Autodesk Fusion 360 part; units mm, degrees
(part 2 of 7)
  spline S21 degree 5 poles (-29.1022, 12.0545) (-29.1083, 12.0397) (-29.1203, 12.01) (-29.1375, 11.9653) (-29.159, 11.9055) (-29.1833, 11.8303) (-29.2052, 11.7547) (-29.2246, 11.6787) (-29.2416, 11.6024) (-29.256, 11.5259) (-29.268, 11.4493) (-29.2775, 11.3726) (-29.2844, 11.2962) (-29.2889, 11.22) (-29.2909, 11.1444) (-29.2905, 11.0694) (-29.2877, 10.9953) (-29.2826, 10.9223) (-29.2753, 10.8505) (-29.2659, 10.7801) (-29.2545, 10.7112) (-29.2411, 10.6438) (-29.2258, 10.5781) (-29.2087, 10.5142) (-29.1899, 10.452) (-29.1695, 10.3917) (-29.1478, 10.3334) (-29.125, 10.2775) (-29.1013, 10.2243) (-29.0773, 10.1741) (-29.0531, 10.127) (-29.0289, 10.0831) (-29.005, 10.042) (-28.9815, 10.0035) (-28.9585, 9.967) (-28.9365, 9.9326) (-28.9164, 9.9006) (-28.8995, 9.8722) (-28.8873, 9.8487) (-28.8804, 9.8308) (-28.8783, 9.8185) (-28.8793, 9.8102) (-28.8813, 9.8039) (-28.8835, 9.7977) (-28.8879, 9.7905) (-28.897, 9.7819) (-28.9133, 9.772) (-28.9374, 9.7607) (-28.968, 9.7485) (-29.0034, 9.7354) (-29.0418, 9.7214) (-29.0823, 9.7065) (-29.1244, 9.6903) (-29.1684, 9.6723) (-29.2143, 9.6521) (-29.2622, 9.6295) (-29.3118, 9.6043) (-29.363, 9.5764) (-29.4151, 9.546) (-29.4678, 9.513) (-29.5206, 9.4776) (-29.5734, 9.4397) (-29.6259, 9.3993) (-29.678, 9.3565) (-29.7297, 9.3112) (-29.7807, 9.2635) (-29.8311, 9.2134) (-29.8806, 9.1609) (-29.9291, 9.1061) (-29.9764, 9.049) (-30.0223, 8.9898) (-30.0668, 8.9285) (-30.1096, 8.8654) (-30.1506, 8.8005) (-30.1898, 8.7339) (-30.2269, 8.6658) (-30.262, 8.5963) (-30.295, 8.5255) (-30.3258, 8.4534) (-30.3545, 8.3801) (-30.3809, 8.3056) (-30.4003, 8.2451) (-30.4139, 8.1991) (-30.4225, 8.1683) (-30.4267, 8.1528) knots 0 0 0 0 0 0 0.0125 0.025 0.0375 0.05 0.0625 0.075 0.0875 0.1 0.1125 0.125 0.1375 0.15 0.1625 0.175 0.1875 0.2 0.2125 0.225 0.2375 0.25 0.2625 0.275 0.2875 0.3 0.3125 0.325 0.3375 0.35 0.3625 0.375 0.3875 0.4 0.4125 0.425 0.4375 0.45 0.4625 0.475 0.4875 0.5 0.5125 0.525 0.5375 0.55 0.5625 0.575 0.5875 0.6 0.6125 0.625 0.6375 0.65 0.6625 0.675 0.6875 0.7 0.7125 0.725 0.7375 0.75 0.7625 0.775 0.7875 0.8 0.8125 0.825 0.8375 0.85 0.8625 0.875 0.8875 0.9 0.9125 0.925 0.9375 0.95 0.9625 0.975 0.9875 1 1 1 1 1 1
  spline S22 degree 5 poles (-30.4267, 8.1528) (-30.4308, 8.1373) (-30.4388, 8.1063) (-30.45, 8.0597) (-30.4635, 7.9976) (-30.4778, 7.9199) (-30.4897, 7.8421) (-30.499, 7.7642) (-30.5058, 7.6864) (-30.5102, 7.6086) (-30.512, 7.5311) (-30.5114, 7.4539) (-30.5083, 7.3771) (-30.5028, 7.301) (-30.495, 7.2258) (-30.4848, 7.1515) (-30.4723, 7.0785) (-30.4578, 7.0067) (-30.4412, 6.9365) (-30.4226, 6.8679) (-30.4023, 6.8011) (-30.3802, 6.736) (-30.3565, 6.6729) (-30.3312, 6.6117) (-30.3044, 6.5525) (-30.2764, 6.4954) (-30.2472, 6.4405) (-30.2173, 6.388) (-30.1869, 6.3384) (-30.1565, 6.2917) (-30.1263, 6.2482) (-30.0967, 6.2078) (-30.0676, 6.1702) (-30.0393, 6.135) (-30.0117, 6.1019) (-29.9854, 6.0706) (-29.9613, 6.0416) (-29.9409, 6.0156) (-29.9256, 5.9939) (-29.9165, 5.9771) (-29.9129, 5.9651) (-29.9127, 5.9568) (-29.9139, 5.9502) (-29.9153, 5.9438) (-29.9186, 5.9361) (-29.9265, 5.9264) (-29.9415, 5.9144) (-29.9638, 5.9001) (-29.9926, 5.884) (-30.026, 5.8664) (-30.0623, 5.8476) (-30.1004, 5.8275) (-30.1401, 5.8059) (-30.1813, 5.7823) (-30.2242, 5.7563) (-30.2687, 5.7276) (-30.3147, 5.6961) (-30.3617, 5.6619) (-30.4094, 5.6249) (-30.4574, 5.5853) (-30.5052, 5.5433) (-30.5525, 5.4988) (-30.5993, 5.4519) (-30.6454, 5.4027) (-30.6907, 5.3511) (-30.7351, 5.2971) (-30.7785, 5.2408) (-30.8207, 5.1823) (-30.8616, 5.1216) (-30.9011, 5.0589) (-30.9389, 4.9942) (-30.975, 4.9277) (-31.0092, 4.8595) (-31.0414, 4.7897) (-31.0715, 4.7186) (-31.0994, 4.6463) (-31.1252, 4.5728) (-31.1486, 4.4983) (-31.1698, 4.4228) (-31.1886, 4.3463) (-31.2051, 4.269) (-31.2164, 4.2065) (-31.2239, 4.1592) (-31.2284, 4.1275) (-31.2305, 4.1116) knots 0 0 0 0 0 0 0.0125 0.025 0.0375 0.05 0.0625 0.075 0.0875 0.1 0.1125 0.125 0.1375 0.15 0.1625 0.175 0.1875 0.2 0.2125 0.225 0.2375 0.25 0.2625 0.275 0.2875 0.3 0.3125 0.325 0.3375 0.35 0.3625 0.375 0.3875 0.4 0.4125 0.425 0.4375 0.45 0.4625 0.475 0.4875 0.5 0.5125 0.525 0.5375 0.55 0.5625 0.575 0.5875 0.6 0.6125 0.625 0.6375 0.65 0.6625 0.675 0.6875 0.7 0.7125 0.725 0.7375 0.75 0.7625 0.775 0.7875 0.8 0.8125 0.825 0.8375 0.85 0.8625 0.875 0.8875 0.9 0.9125 0.925 0.9375 0.95 0.9625 0.975 0.9875 1 1 1 1 1 1
  spline S23 degree 5 poles (-31.2305, 4.1116) (-31.2326, 4.0957) (-31.2364, 4.0639) (-31.2415, 4.0163) (-31.2467, 3.9529) (-31.2508, 3.874) (-31.2524, 3.7953) (-31.2515, 3.7169) (-31.2481, 3.6388) (-31.2423, 3.5612) (-31.234, 3.484) (-31.2233, 3.4076) (-31.2102, 3.3319) (-31.1949, 3.2572) (-31.1772, 3.1836) (-31.1574, 3.1113) (-31.1356, 3.0405) (-31.1118, 2.9713) (-31.0861, 2.9038) (-31.0588, 2.8382) (-31.0299, 2.7746) (-30.9995, 2.713) (-30.9678, 2.6535) (-30.9347, 2.5961) (-30.9004, 2.5409) (-30.8651, 2.4879) (-30.8291, 2.4373) (-30.7926, 2.3893) (-30.756, 2.344) (-30.7197, 2.3017) (-30.6842, 2.2624) (-30.6495, 2.2262) (-30.6158, 2.1928) (-30.583, 2.1616) (-30.5514, 2.1324) (-30.5212, 2.1048) (-30.4935, 2.0792) (-30.4699, 2.0561) (-30.452, 2.0365) (-30.4407, 2.0211) (-30.4356, 2.0097) (-30.4343, 2.0014) (-30.4346, 1.9948) (-30.4352, 1.9882) (-30.4375, 1.9801) (-30.4441, 1.9695) (-30.4573, 1.9557) (-30.4776, 1.9386) (-30.504, 1.9188) (-30.5348, 1.897) (-30.5683, 1.8736) (-30.6036, 1.8487) (-30.6401, 1.8221) (-30.6779, 1.7934) (-30.717, 1.762) (-30.7574, 1.7278) (-30.7988, 1.6905) (-30.841, 1.6504) (-30.8835, 1.6075) (-30.9258, 1.5621) (-30.9677, 1.5141) (-31.0089, 1.4639) (-31.0492, 1.4113) (-31.0884, 1.3565) (-31.1266, 1.2994) (-31.1636, 1.2401) (-31.1992, 1.1786) (-31.2334, 1.1151) (-31.2661, 1.0496) (-31.297, 0.9822) (-31.3261, 0.9131) (-31.3532, 0.8424) (-31.3782, 0.7704) (-31.401, 0.6971) (-31.4216, 0.6226) (-31.4398, 0.5472) (-31.4558, 0.471) (-31.4693, 0.3941) (-31.4804, 0.3164) (-31.4891, 0.2382) (-31.4954, 0.1594) (-31.4984, 0.0959) (-31.4996, 0.0481) (-31.5, 0.016) (-31.5, 0) knots 0 0 0 0 0 0 0.0125 0.025 0.0375 0.05 0.0625 0.075 0.0875 0.1 0.1125 0.125 0.1375 0.15 0.1625 0.175 0.1875 0.2 0.2125 0.225 0.2375 0.25 0.2625 0.275 0.2875 0.3 0.3125 0.325 0.3375 0.35 0.3625 0.375 0.3875 0.4 0.4125 0.425 0.4375 0.45 0.4625 0.475 0.4875 0.5 0.5125 0.525 0.5375 0.55 0.5625 0.575 0.5875 0.6 0.6125 0.625 0.6375 0.65 0.6625 0.675 0.6875 0.7 0.7125 0.725 0.7375 0.75 0.7625 0.775 0.7875 0.8 0.8125 0.825 0.8375 0.85 0.8625 0.875 0.8875 0.9 0.9125 0.925 0.9375 0.95 0.9625 0.975 0.9875 1 1 1 1 1 1
  spline S24 degree 5 poles (-31.5, 0) (-31.5, -0.016) (-31.4996, -0.0481) (-31.4984, -0.0959) (-31.4954, -0.1594) (-31.4891, -0.2382) (-31.4804, -0.3164) (-31.4693, -0.3941) (-31.4558, -0.471) (-31.4398, -0.5472) (-31.4216, -0.6226) (-31.401, -0.697) (-31.3781, -0.7704) (-31.3531, -0.8424) (-31.326, -0.9131) (-31.297, -0.9822) (-31.266, -1.0496) (-31.2334, -1.1151) (-31.1992, -1.1786) (-31.1636, -1.2401) (-31.1266, -1.2994) (-31.0884, -1.3565) (-31.0492, -1.4113) (-31.0089, -1.4639) (-30.9677, -1.5141) (-30.9258, -1.5621) (-30.8835, -1.6075) (-30.841, -1.6504) (-30.7988, -1.6906) (-30.7574, -1.7278) (-30.717, -1.762) (-30.6779, -1.7934) (-30.6401, -1.8221) (-30.6036, -1.8487) (-30.5683, -1.8736) (-30.5348, -1.897) (-30.504, -1.9188) (-30.4776, -1.9386) (-30.4573, -1.9557) (-30.4441, -1.9695) (-30.4375, -1.9801) (-30.4352, -1.9882) (-30.4346, -1.9948) (-30.4343, -2.0014) (-30.4356, -2.0097) (-30.4407, -2.0211) (-30.452, -2.0365) (-30.4699, -2.0561) (-30.4935, -2.0792) (-30.5212, -2.1048) (-30.5514, -2.1324) (-30.583, -2.1616) (-30.6158, -2.1928) (-30.6495, -2.2262) (-30.6842, -2.2624) (-30.7197, -2.3017) (-30.756, -2.344) (-30.7926, -2.3893) (-30.8291, -2.4373) (-30.8652, -2.4879) (-30.9004, -2.5409) (-30.9347, -2.5961) (-30.9677, -2.6535) (-30.9995, -2.713) (-31.0299, -2.7746) (-31.0588, -2.8382) (-31.0862, -2.9038) (-31.1118, -2.9713) (-31.1356, -3.0405) (-31.1575, -3.1113) (-31.1773, -3.1836) (-31.1949, -3.2572) (-31.2103, -3.3319) (-31.2233, -3.4076) (-31.234, -3.484) (-31.2423, -3.5612) (-31.2481, -3.6388) (-31.2515, -3.7169) (-31.2524, -3.7953) (-31.2508, -3.874) (-31.2467, -3.9529) (-31.2415, -4.0163) (-31.2364, -4.0639) (-31.2326, -4.0957) (-31.2305, -4.1116) knots 0 0 0 0 0 0 0.0125 0.025 0.0375 0.05 0.0625 0.075 0.0875 0.1 0.1125 0.125 0.1375 0.15 0.1625 0.175 0.1875 0.2 0.2125 0.225 0.2375 0.25 0.2625 0.275 0.2875 0.3 0.3125 0.325 0.3375 0.35 0.3625 0.375 0.3875 0.4 0.4125 0.425 0.4375 0.45 0.4625 0.475 0.4875 0.5 0.5125 0.525 0.5375 0.55 0.5625 0.575 0.5875 0.6 0.6125 0.625 0.6375 0.65 0.6625 0.675 0.6875 0.7 0.7125 0.725 0.7375 0.75 0.7625 0.775 0.7875 0.8 0.8125 0.825 0.8375 0.85 0.8625 0.875 0.8875 0.9 0.9125 0.925 0.9375 0.95 0.9625 0.975 0.9875 1 1 1 1 1 1
  spline S25 degree 5 poles (-31.2305, -4.1116) (-31.2284, -4.1275) (-31.2239, -4.1592) (-31.2165, -4.2065) (-31.2051, -4.269) (-31.1886, -4.3463) (-31.1698, -4.4228) (-31.1486, -4.4983) (-31.1252, -4.5728) (-31.0994, -4.6463) (-31.0715, -4.7186) (-31.0413, -4.7897) (-31.0091, -4.8595) (-30.9749, -4.9276) (-30.9389, -4.9942) (-30.901, -5.0589) (-30.8616, -5.1216) (-30.8207, -5.1823) (-30.7785, -5.2408) (-30.7351, -5.2971) (-30.6907, -5.3511) (-30.6454, -5.4027) (-30.5993, -5.452) (-30.5525, -5.4988) (-30.5052, -5.5433) (-30.4574, -5.5853) (-30.4094, -5.6249) (-30.3617, -5.6619) (-30.3147, -5.6961) (-30.2687, -5.7276) (-30.2242, -5.7563) (-30.1813, -5.7823) (-30.1401, -5.8059) (-30.1004, -5.8275) (-30.0623, -5.8476) (-30.026, -5.8664) (-29.9926, -5.884) (-29.9638, -5.9001) (-29.9415, -5.9144) (-29.9265, -5.9264) (-29.9186, -5.9361) (-29.9153, -5.9438) (-29.9139, -5.9502) (-29.9127, -5.9568) (-29.9129, -5.9651) (-29.9165, -5.9771) (-29.9257, -5.9939) (-29.9409, -6.0156) (-29.9613, -6.0416) (-29.9854, -6.0706) (-30.0117, -6.1019) (-30.0393, -6.135) (-30.0676, -6.1702) (-30.0967, -6.2078) (-30.1263, -6.2482) (-30.1565, -6.2917) (-30.1869, -6.3384) (-30.2173, -6.3881) (-30.2472, -6.4405) (-30.2764, -6.4954) (-30.3044, -6.5525) (-30.3312, -6.6117) (-30.3565, -6.6729) (-30.3802, -6.736) (-30.4023, -6.8011) (-30.4226, -6.8679) (-30.4412, -6.9365) (-30.4578, -7.0067) (-30.4724, -7.0785) (-30.4848, -7.1515) (-30.495, -7.2258) (-30.5029, -7.3011) (-30.5084, -7.3771) (-30.5115, -7.4539) (-30.5121, -7.5311) (-30.5102, -7.6086) (-30.5058, -7.6864) (-30.499, -7.7642) (-30.4896, -7.8421) (-30.4778, -7.9199) (-30.4634, -7.9976) (-30.45, -8.0597) (-30.4388, -8.1063) (-30.4308, -8.1373) (-30.4267, -8.1528) knots 0 0 0 0 0 0 0.0125 0.025 0.0375 0.05 0.0625 0.075 0.0875 0.1 0.1125 0.125 0.1375 0.15 0.1625 0.175 0.1875 0.2 0.2125 0.225 0.2375 0.25 0.2625 0.275 0.2875 0.3 0.3125 0.325 0.3375 0.35 0.3625 0.375 0.3875 0.4 0.4125 0.425 0.4375 0.45 0.4625 0.475 0.4875 0.5 0.5125 0.525 0.5375 0.55 0.5625 0.575 0.5875 0.6 0.6125 0.625 0.6375 0.65 0.6625 0.675 0.6875 0.7 0.7125 0.725 0.7375 0.75 0.7625 0.775 0.7875 0.8 0.8125 0.825 0.8375 0.85 0.8625 0.875 0.8875 0.9 0.9125 0.925 0.9375 0.95 0.9625 0.975 0.9875 1 1 1 1 1 1
  spline S26 degree 5 poles (-30.4267, -8.1528) (-30.4225, -8.1683) (-30.4139, -8.1991) (-30.4003, -8.2451) (-30.3809, -8.3056) (-30.3545, -8.3801) (-30.3259, -8.4534) (-30.295, -8.5255) (-30.262, -8.5963) (-30.2269, -8.6658) (-30.1897, -8.7339) (-30.1506, -8.8005) (-30.1096, -8.8654) (-30.0668, -8.9285) (-30.0223, -8.9898) (-29.9763, -9.049) (-29.929, -9.106) (-29.8806, -9.1609) (-29.8311, -9.2134) (-29.7807, -9.2635) (-29.7297, -9.3113) (-29.678, -9.3565) (-29.6259, -9.3993) (-29.5734, -9.4397) (-29.5206, -9.4776) (-29.4678, -9.513) (-29.4151, -9.546) (-29.363, -9.5764) (-29.3118, -9.6043) (-29.2621, -9.6295) (-29.2143, -9.6521) (-29.1684, -9.6723) (-29.1244, -9.6903) (-29.0823, -9.7065) (-29.0418, -9.7214) (-29.0034, -9.7354) (-28.968, -9.7485) (-28.9374, -9.7607) (-28.9133, -9.772) (-28.897, -9.7819) (-28.8879, -9.7905) (-28.8835, -9.7977) (-28.8813, -9.8039) (-28.8793, -9.8102) (-28.8783, -9.8185) (-28.8804, -9.8308) (-28.8873, -9.8487) (-28.8995, -9.8722) (-28.9164, -9.9006) (-28.9365, -9.9326) (-28.9585, -9.967) (-28.9815, -10.0035) (-29.005, -10.042) (-29.0289, -10.0831) (-29.0531, -10.127) (-29.0773, -10.1741) (-29.1014, -10.2243) (-29.125, -10.2775) (-29.1478, -10.3334) (-29.1695, -10.3917) (-29.1899, -10.452) (-29.2087, -10.5142) (-29.2258, -10.5781) (-29.2411, -10.6438) (-29.2545, -10.7112) (-29.2659, -10.7801) (-29.2754, -10.8505) (-29.2827, -10.9223) (-29.2878, -10.9954) (-29.2905, -11.0694) (-29.291, -11.1444) (-29.289, -11.22) (-29.2845, -11.2962) (-29.2775, -11.3727) (-29.268, -11.4493) (-29.256, -11.5259) (-29.2416, -11.6024) (-29.2246, -11.6787) (-29.2052, -11.7547) (-29.1833, -11.8303) (-29.1589, -11.9055) (-29.1375, -11.9653) (-29.1203, -12.01) (-29.1083, -12.0397) (-29.1022, -12.0545) knots 0 0 0 0 0 0 0.0125 0.025 0.0375 0.05 0.0625 0.075 0.0875 0.1 0.1125 0.125 0.1375 0.15 0.1625 0.175 0.1875 0.2 0.2125 0.225 0.2375 0.25 0.2625 0.275 0.2875 0.3 0.3125 0.325 0.3375 0.35 0.3625 0.375 0.3875 0.4 0.4125 0.425 0.4375 0.45 0.4625 0.475 0.4875 0.5 0.5125 0.525 0.5375 0.55 0.5625 0.575 0.5875 0.6 0.6125 0.625 0.6375 0.65 0.6625 0.675 0.6875 0.7 0.7125 0.725 0.7375 0.75 0.7625 0.775 0.7875 0.8 0.8125 0.825 0.8375 0.85 0.8625 0.875 0.8875 0.9 0.9125 0.925 0.9375 0.95 0.9625 0.975 0.9875 1 1 1 1 1 1
  spline S27 degree 5 poles (-29.1022, -12.0545) (-29.096, -12.0693) (-29.0835, -12.0988) (-29.0641, -12.1426) (-29.0369, -12.2001) (-29.001, -12.2705) (-28.963, -12.3394) (-28.923, -12.4068) (-28.8811, -12.4728) (-28.8372, -12.5371) (-28.7915, -12.5997) (-28.744, -12.6606) (-28.6948, -12.7196) (-28.6441, -12.7766) (-28.5921, -12.8315) (-28.5388, -12.8842) (-28.4844, -12.9347) (-28.4292, -12.9827) (-28.3733, -13.0283) (-28.3168, -13.0714) (-28.26, -13.1121) (-28.2029, -13.1502) (-28.1456, -13.1859) (-28.0883, -13.219) (-28.031, -13.2497) (-27.974, -13.278) (-27.9174, -13.3038) (-27.8618, -13.3271) (-27.8075, -13.3481) (-27.7549, -13.3666) (-27.7045, -13.3828) (-27.6564, -13.3968) (-27.6104, -13.4089) (-27.5665, -13.4195) (-27.5245, -13.429) (-27.4846, -13.4378) (-27.4477, -13.4462) (-27.4158, -13.4543) (-27.3905, -13.4623) (-27.373, -13.47) (-27.3628, -13.4773) (-27.3576, -13.4839) (-27.3545, -13.4898) (-27.3517, -13.4958) (-27.3497, -13.5039) (-27.3501, -13.5164) (-27.3546, -13.535) (-27.3637, -13.5599) (-27.3767, -13.5903) (-27.3924, -13.6246) (-27.4098, -13.6616) (-27.4278, -13.7007) (-27.4462, -13.742) (-27.4645, -13.7858) (-27.4827, -13.8325) (-27.5005, -13.8824) (-27.5178, -13.9354) (-27.5343, -13.9912) (-27.5496, -14.0496) (-27.5636, -14.1101) (-27.5759, -14.1726) (-27.5864, -14.2367) (-27.595, -14.3024) (-27.6016, -14.3695) (-27.6061, -14.438) (-27.6085, -14.5079) (-27.6086, -14.5789) (-27.6065, -14.651) (-27.602, -14.7241) (-27.5951, -14.7979) (-27.5857, -14.8723) (-27.5739, -14.947) (-27.5595, -15.0219) (-27.5426, -15.0968) (-27.5232, -15.1716) (-27.5013, -15.246) (-27.477, -15.32) (-27.4502, -15.3934) (-27.4211, -15.4662) (-27.3895, -15.5382) (-27.3555, -15.6096) (-27.3264, -15.6661) (-27.3035, -15.7082) (-27.2878, -15.7361) (-27.2798, -15.75) knots 0 0 0 0 0 0 0.0125 0.025 0.0375 0.05 0.0625 0.075 0.0875 0.1 0.1125 0.125 0.1375 0.15 0.1625 0.175 0.1875 0.2 0.2125 0.225 0.2375 0.25 0.2625 0.275 0.2875 0.3 0.3125 0.325 0.3375 0.35 0.3625 0.375 0.3875 0.4 0.4125 0.425 0.4375 0.45 0.4625 0.475 0.4875 0.5 0.5125 0.525 0.5375 0.55 0.5625 0.575 0.5875 0.6 0.6125 0.625 0.6375 0.65 0.6625 0.675 0.6875 0.7 0.7125 0.725 0.7375 0.75 0.7625 0.775 0.7875 0.8 0.8125 0.825 0.8375 0.85 0.8625 0.875 0.8875 0.9 0.9125 0.925 0.9375 0.95 0.9625 0.975 0.9875 1 1 1 1 1 1
  spline S28 degree 5 poles (-27.2798, -15.75) (-27.2717, -15.7639) (-27.2555, -15.7915) (-27.2305, -15.8323) (-27.1961, -15.8858) (-27.1513, -15.9509) (-27.1046, -16.0143) (-27.0562, -16.0759) (-27.006, -16.1358) (-26.9541, -16.1938) (-26.9006, -16.25) (-26.8455, -16.3041) (-26.7891, -16.3562) (-26.7314, -16.4061) (-26.6726, -16.4538) (-26.6129, -16.4991) (-26.5524, -16.542) (-26.4914, -16.5824) (-26.43, -16.6203) (-26.3684, -16.6557) (-26.3067, -16.6886) (-26.2451, -16.7189) (-26.1837, -16.7468) (-26.1226, -16.7722) (-26.0618, -16.7951) (-26.0015, -16.8157) (-25.9421, -16.8339) (-25.8839, -16.8498) (-25.8273, -16.8635) (-25.7728, -16.875) (-25.7207, -16.8844) (-25.6711, -16.892) (-25.624, -16.8981) (-25.5791, -16.9028) (-25.5362, -16.9068) (-25.4954, -16.9103) (-25.4578, -16.9138) (-25.4251, -16.9177) (-25.399, -16.9223) (-25.3806, -16.9277) (-25.3696, -16.9336) (-25.3635, -16.9394) (-25.3597, -16.9448) (-25.3562, -16.9504) (-25.3531, -16.9582) (-25.3519, -16.9707) (-25.3539, -16.9897) (-25.3597, -17.0156) (-25.3686, -17.0474) (-25.3797, -17.0834) (-25.3921, -17.1224) (-25.4049, -17.1636) (-25.4177, -17.2069) (-25.4301, -17.2527) (-25.442, -17.3014) (-25.4532, -17.3532) (-25.4635, -17.4079) (-25.4725, -17.4654) (-25.4801, -17.5253) (-25.486, -17.5872) (-25.4901, -17.6507) (-25.4921, -17.7157) (-25.4921, -17.7819) (-25.4899, -17.8493) (-25.4854, -17.9178) (-25.4786, -17.9874) (-25.4695, -18.0578) (-25.458, -18.1291) (-25.444, -18.2009) (-25.4275, -18.2732) (-25.4085, -18.3457) (-25.387, -18.4182) (-25.363, -18.4906) (-25.3364, -18.5627) (-25.3074, -18.6343) (-25.276, -18.7052) (-25.2423, -18.7754) (-25.2061, -18.8447) (-25.1677, -18.913) (-25.127, -18.9804) (-25.084, -19.0467) (-25.0478, -19.0989) (-25.0196, -19.1376) (-25.0004, -19.1632) (-24.9906, -19.176) knots 0 0 0 0 0 0 0.0125 0.025 0.0375 0.05 0.0625 0.075 0.0875 0.1 0.1125 0.125 0.1375 0.15 0.1625 0.175 0.1875 0.2 0.2125 0.225 0.2375 0.25 0.2625 0.275 0.2875 0.3 0.3125 0.325 0.3375 0.35 0.3625 0.375 0.3875 0.4 0.4125 0.425 0.4375 0.45 0.4625 0.475 0.4875 0.5 0.5125 0.525 0.5375 0.55 0.5625 0.575 0.5875 0.6 0.6125 0.625 0.6375 0.65 0.6625 0.675 0.6875 0.7 0.7125 0.725 0.7375 0.75 0.7625 0.775 0.7875 0.8 0.8125 0.825 0.8375 0.85 0.8625 0.875 0.8875 0.9 0.9125 0.925 0.9375 0.95 0.9625 0.975 0.9875 1 1 1 1 1 1
  spline S29 degree 5 poles (-24.9906, -19.176) (-24.9808, -19.1887) (-24.9611, -19.2139) (-24.931, -19.2512) (-24.8899, -19.2997) (-24.837, -19.3584) (-24.7825, -19.4151) (-24.7264, -19.4699) (-24.6688, -19.5227) (-24.6098, -19.5735) (-24.5494, -19.6222) (-24.4877, -19.6687) (-24.425, -19.713) (-24.3613, -19.7549) (-24.2968, -19.7945) (-24.2316, -19.8316) (-24.1661, -19.8662) (-24.1003, -19.8983) (-24.0345, -19.9279) (-23.9688, -19.955) (-23.9034, -19.9795) (-23.8384, -20.0016) (-23.7738, -20.0212) (-23.7099, -20.0384) (-23.6466, -20.0532) (-23.5842, -20.0657) (-23.5229, -20.076) (-23.4631, -20.0842) (-23.4052, -20.0903) (-23.3497, -20.0946) (-23.2968, -20.0972) (-23.2466, -20.0983) (-23.1992, -20.0981) (-23.154, -20.097) (-23.1109, -20.0953) (-23.0701, -20.0934) (-23.0324, -20.092) (-22.9994, -20.0916) (-22.9729, -20.0928) (-22.9539, -20.0957) (-22.9422, -20.1001) (-22.9355, -20.1051) (-22.931, -20.11) (-22.9268, -20.1151) (-22.9227, -20.1224) (-22.9199, -20.1346) (-22.9194, -20.1537) (-22.9217, -20.1801) (-22.9264, -20.2128) (-22.9328, -20.25) (-22.9399, -20.2902) (-22.9472, -20.3327) (-22.9542, -20.3774) (-22.9606, -20.4244) (-22.9661, -20.4742) (-22.9704, -20.527) (-22.9735, -20.5827) (-22.9749, -20.6409) (-22.9746, -20.7012) (-22.9724, -20.7633) (-22.9681, -20.8268) (-22.9617, -20.8915) (-22.953, -20.9571) (-22.942, -21.0237) (-22.9286, -21.091) (-22.9128, -21.1591) (-22.8946, -21.2278) (-22.8739, -21.2969) (-22.8506, -21.3663) (-22.8248, -21.4358) (-22.7966, -21.5052) (-22.7657, -21.5743) (-22.7325, -21.643) (-22.6968, -21.711) (-22.6587, -21.7782) (-22.6183, -21.8444) (-22.5756, -21.9095) (-22.5308, -21.9735) (-22.4838, -22.0362) (-22.4346, -22.0977) (-22.3833, -22.1579) (-22.3406, -22.2049) (-22.3076, -22.2396) (-22.2852, -22.2625) (-22.2739, -22.2739) knots 0 0 0 0 0 0 0.0125 0.025 0.0375 0.05 0.0625 0.075 0.0875 0.1 0.1125 0.125 0.1375 0.15 0.1625 0.175 0.1875 0.2 0.2125 0.225 0.2375 0.25 0.2625 0.275 0.2875 0.3 0.3125 0.325 0.3375 0.35 0.3625 0.375 0.3875 0.4 0.4125 0.425 0.4375 0.45 0.4625 0.475 0.4875 0.5 0.5125 0.525 0.5375 0.55 0.5625 0.575 0.5875 0.6 0.6125 0.625 0.6375 0.65 0.6625 0.675 0.6875 0.7 0.7125 0.725 0.7375 0.75 0.7625 0.775 0.7875 0.8 0.8125 0.825 0.8375 0.85 0.8625 0.875 0.8875 0.9 0.9125 0.925 0.9375 0.95 0.9625 0.975 0.9875 1 1 1 1 1 1
  spline S30 degree 5 poles (-22.2739, -22.2739) (-22.2625, -22.2852) (-22.2396, -22.3076) (-22.2049, -22.3406) (-22.1579, -22.3833) (-22.0977, -22.4346) (-22.0363, -22.4838) (-21.9735, -22.5308) (-21.9095, -22.5756) (-21.8444, -22.6183) (-21.7781, -22.6587) (-21.7109, -22.6967) (-21.643, -22.7324) (-21.5743, -22.7657) (-21.5052, -22.7965) (-21.4358, -22.8248) (-21.3663, -22.8506) (-21.2969, -22.8738) (-21.2278, -22.8946) (-21.1591, -22.9128) (-21.091, -22.9286) (-21.0237, -22.942) (-20.9571, -22.953) (-20.8915, -22.9617) (-20.8268, -22.9681) (-20.7633, -22.9724) (-20.7012, -22.9746) (-20.6409, -22.9749) (-20.5827, -22.9735) (-20.527, -22.9704) (-20.4742, -22.9661) (-20.4244, -22.9606) (-20.3774, -22.9542) (-20.3327, -22.9472) (-20.2902, -22.9399) (-20.25, -22.9328) (-20.2128, -22.9264) (-20.1801, -22.9217) (-20.1537, -22.9194) (-20.1345, -22.9199) (-20.1224, -22.9227) (-20.1151, -22.9268) (-20.11, -22.931) (-20.1051, -22.9355) (-20.1001, -22.9422) (-20.0957, -22.9539) (-20.0928, -22.9729) (-20.0916, -22.9994) (-20.092, -23.0324) (-20.0934, -23.0701) (-20.0953, -23.1109) (-20.097, -23.154) (-20.0981, -23.1992) (-20.0983, -23.2467) (-20.0972, -23.2968) (-20.0946, -23.3497) (-20.0903, -23.4052) (-20.0842, -23.4631) (-20.076, -23.5229) (-20.0657, -23.5842) (-20.0532, -23.6466) (-20.0384, -23.7099) (-20.0212, -23.7738) (-20.0016, -23.8384) (-19.9795, -23.9034) (-19.955, -23.9688) (-19.9279, -24.0345) (-19.8984, -24.1004) (-19.8663, -24.1661) (-19.8316, -24.2317) (-19.7945, -24.2968) (-19.755, -24.3613) (-19.713, -24.425) (-19.6687, -24.4878) (-19.6222, -24.5494) (-19.5735, -24.6098) (-19.5227, -24.6688) (-19.4699, -24.7264) (-19.4151, -24.7824) (-19.3583, -24.837) (-19.2996, -24.8899) (-19.2511, -24.931) (-19.2139, -24.9611) (-19.1887, -24.9808) (-19.176, -24.9906) knots 0 0 0 0 0 0 0.0125 0.025 0.0375 0.05 0.0625 0.075 0.0875 0.1 0.1125 0.125 0.1375 0.15 0.1625 0.175 0.1875 0.2 0.2125 0.225 0.2375 0.25 0.2625 0.275 0.2875 0.3 0.3125 0.325 0.3375 0.35 0.3625 0.375 0.3875 0.4 0.4125 0.425 0.4375 0.45 0.4625 0.475 0.4875 0.5 0.5125 0.525 0.5375 0.55 0.5625 0.575 0.5875 0.6 0.6125 0.625 0.6375 0.65 0.6625 0.675 0.6875 0.7 0.7125 0.725 0.7375 0.75 0.7625 0.775 0.7875 0.8 0.8125 0.825 0.8375 0.85 0.8625 0.875 0.8875 0.9 0.9125 0.925 0.9375 0.95 0.9625 0.975 0.9875 1 1 1 1 1 1
  spline S31 degree 5 poles (-19.176, -24.9906) (-19.1632, -25.0004) (-19.1376, -25.0196) (-19.0989, -25.0478) (-19.0467, -25.084) (-18.9804, -25.127) (-18.913, -25.1677) (-18.8447, -25.2062) (-18.7754, -25.2423) (-18.7052, -25.276) (-18.6343, -25.3074) (-18.5627, -25.3364) (-18.4906, -25.3629) (-18.4182, -25.387) (-18.3457, -25.4085) (-18.2732, -25.4275) (-18.2009, -25.444) (-18.1291, -25.4579) (-18.0578, -25.4695) (-17.9874, -25.4786) (-17.9178, -25.4854) (-17.8493, -25.4899) (-17.7819, -25.4921) (-17.7157, -25.4922) (-17.6507, -25.4901) (-17.5872, -25.486) (-17.5253, -25.4801) (-17.4654, -25.4725) (-17.4079, -25.4635) (-17.3532, -25.4532) (-17.3014, -25.442) (-17.2527, -25.4301) (-17.2069, -25.4177) (-17.1636, -25.4049) (-17.1224, -25.3921) (-17.0834, -25.3797) (-17.0474, -25.3686) (-17.0156, -25.3597) (-16.9897, -25.3539) (-16.9707, -25.3519) (-16.9582, -25.3531) (-16.9504, -25.3562) (-16.9448, -25.3597) (-16.9394, -25.3635) (-16.9336, -25.3696) (-16.9277, -25.3806) (-16.9223, -25.399) (-16.9177, -25.4251) (-16.9138, -25.4578) (-16.9103, -25.4954) (-16.9068, -25.5362) (-16.9028, -25.5791) (-16.898, -25.624) (-16.892, -25.6711) (-16.8844, -25.7207) (-16.875, -25.7728) (-16.8635, -25.8273) (-16.8498, -25.8839) (-16.8339, -25.9421) (-16.8157, -26.0015) (-16.7951, -26.0618) (-16.7722, -26.1226) (-16.7468, -26.1837) (-16.7189, -26.2451) (-16.6886, -26.3067) (-16.6557, -26.3684) (-16.6203, -26.43) (-16.5824, -26.4914) (-16.542, -26.5525) (-16.4991, -26.6129) (-16.4538, -26.6726) (-16.4062, -26.7314) (-16.3563, -26.7891) (-16.3042, -26.8455) (-16.25, -26.9006) (-16.1938, -26.9541) (-16.1358, -27.006) (-16.0759, -27.0562) (-16.0143, -27.1046) (-15.9509, -27.1512) (-15.8857, -27.1961) (-15.8323, -27.2305) (-15.7914, -27.2555) (-15.7639, -27.2717) (-15.75, -27.2798) knots 0 0 0 0 0 0 0.0125 0.025 0.0375 0.05 0.0625 0.075 0.0875 0.1 0.1125 0.125 0.1375 0.15 0.1625 0.175 0.1875 0.2 0.2125 0.225 0.2375 0.25 0.2625 0.275 0.2875 0.3 0.3125 0.325 0.3375 0.35 0.3625 0.375 0.3875 0.4 0.4125 0.425 0.4375 0.45 0.4625 0.475 0.4875 0.5 0.5125 0.525 0.5375 0.55 0.5625 0.575 0.5875 0.6 0.6125 0.625 0.6375 0.65 0.6625 0.675 0.6875 0.7 0.7125 0.725 0.7375 0.75 0.7625 0.775 0.7875 0.8 0.8125 0.825 0.8375 0.85 0.8625 0.875 0.8875 0.9 0.9125 0.925 0.9375 0.95 0.9625 0.975 0.9875 1 1 1 1 1 1
  spline S32 degree 5 poles (-15.75, -27.2798) (-15.7361, -27.2878) (-15.7082, -27.3035) (-15.6661, -27.3264) (-15.6096, -27.3555) (-15.5382, -27.3895) (-15.4662, -27.4211) (-15.3934, -27.4502) (-15.32, -27.477) (-15.246, -27.5013) (-15.1716, -27.5232) (-15.0968, -27.5426) (-15.0219, -27.5594) (-14.947, -27.5738) (-14.8722, -27.5857) (-14.7979, -27.5951) (-14.7241, -27.602) (-14.651, -27.6065) (-14.5789, -27.6086) (-14.5078, -27.6085) (-14.438, -27.6061) (-14.3695, -27.6016) (-14.3024, -27.595) (-14.2367, -27.5864) (-14.1726, -27.5759) (-14.1101, -27.5636) (-14.0496, -27.5496) (-13.9912, -27.5343) (-13.9354, -27.5178) (-13.8824, -27.5005) (-13.8325, -27.4827) (-13.7858, -27.4645) (-13.742, -27.4462) (-13.7007, -27.4278) (-13.6616, -27.4098) (-13.6246, -27.3924) (-13.5903, -27.3767) (-13.5599, -27.3637) (-13.535, -27.3546) (-13.5164, -27.3501) (-13.5039, -27.3497) (-13.4958, -27.3517) (-13.4898, -27.3545) (-13.4839, -27.3576) (-13.4773, -27.3628) (-13.47, -27.373) (-13.4623, -27.3905) (-13.4543, -27.4158) (-13.4462, -27.4477) (-13.4378, -27.4846) (-13.429, -27.5245) (-13.4195, -27.5665) (-13.4089, -27.6104) (-13.3968, -27.6564) (-13.3828, -27.7045) (-13.3666, -27.7549) (-13.3481, -27.8075) (-13.3271, -27.8618) (-13.3038, -27.9174) (-13.278, -27.974) (-13.2497, -28.031) (-13.219, -28.0883) (-13.1859, -28.1456) (-13.1502, -28.2029) (-13.1121, -28.26) (-13.0715, -28.3168) (-13.0283, -28.3733) (-12.9827, -28.4292) (-12.9347, -28.4845) (-12.8843, -28.5388) (-12.8316, -28.5921) (-12.7767, -28.6442) (-12.7196, -28.6948) (-12.6606, -28.744) (-12.5997, -28.7915) (-12.5371, -28.8372) (-12.4728, -28.8811) (-12.4068, -28.923) (-12.3394, -28.963) (-12.2704, -29.001) (-12.2, -29.0369) (-12.1426, -29.064) (-12.0988, -29.0835) (-12.0693, -29.096) (-12.0545, -29.1022) knots 0 0 0 0 0 0 0.0125 0.025 0.0375 0.05 0.0625 0.075 0.0875 0.1 0.1125 0.125 0.1375 0.15 0.1625 0.175 0.1875 0.2 0.2125 0.225 0.2375 0.25 0.2625 0.275 0.2875 0.3 0.3125 0.325 0.3375 0.35 0.3625 0.375 0.3875 0.4 0.4125 0.425 0.4375 0.45 0.4625 0.475 0.4875 0.5 0.5125 0.525 0.5375 0.55 0.5625 0.575 0.5875 0.6 0.6125 0.625 0.6375 0.65 0.6625 0.675 0.6875 0.7 0.7125 0.725 0.7375 0.75 0.7625 0.775 0.7875 0.8 0.8125 0.825 0.8375 0.85 0.8625 0.875 0.8875 0.9 0.9125 0.925 0.9375 0.95 0.9625 0.975 0.9875 1 1 1 1 1 1
  spline S33 degree 5 poles (-12.0545, -29.1022) (-12.0397, -29.1083) (-12.01, -29.1203) (-11.9653, -29.1375) (-11.9055, -29.159) (-11.8303, -29.1833) (-11.7547, -29.2052) (-11.6787, -29.2246) (-11.6024, -29.2416) (-11.5259, -29.256) (-11.4493, -29.268) (-11.3726, -29.2775) (-11.2962, -29.2844) (-11.22, -29.2889) (-11.1444, -29.2909) (-11.0694, -29.2905) (-10.9953, -29.2877) (-10.9223, -29.2826) (-10.8505, -29.2753) (-10.7801, -29.2659) (-10.7112, -29.2545) (-10.6438, -29.2411) (-10.5781, -29.2258) (-10.5142, -29.2087) (-10.452, -29.1899) (-10.3917, -29.1695) (-10.3334, -29.1478) (-10.2775, -29.125) (-10.2243, -29.1013) (-10.1741, -29.0773) (-10.127, -29.0531) (-10.0831, -29.0289) (-10.042, -29.005) (-10.0035, -28.9815) (-9.967, -28.9585) (-9.9326, -28.9365) (-9.9006, -28.9164) (-9.8722, -28.8995) (-9.8487, -28.8873) (-9.8308, -28.8804) (-9.8185, -28.8783) (-9.8102, -28.8793) (-9.8039, -28.8813) (-9.7977, -28.8835) (-9.7905, -28.8879) (-9.7819, -28.897) (-9.772, -28.9133) (-9.7607, -28.9374) (-9.7485, -28.968) (-9.7354, -29.0034) (-9.7214, -29.0418) (-9.7065, -29.0823) (-9.6903, -29.1244) (-9.6723, -29.1684) (-9.6521, -29.2143) (-9.6295, -29.2622) (-9.6043, -29.3118) (-9.5764, -29.363) (-9.546, -29.4151) (-9.513, -29.4678) (-9.4776, -29.5206) (-9.4397, -29.5734) (-9.3993, -29.6259) (-9.3565, -29.678) (-9.3112, -29.7297) (-9.2635, -29.7807) (-9.2134, -29.8311) (-9.1609, -29.8806) (-9.1061, -29.9291) (-9.049, -29.9764) (-8.9898, -30.0223) (-8.9285, -30.0668) (-8.8654, -30.1096) (-8.8005, -30.1506) (-8.7339, -30.1898) (-8.6658, -30.2269) (-8.5963, -30.262) (-8.5255, -30.295) (-8.4534, -30.3258) (-8.3801, -30.3545) (-8.3056, -30.3809) (-8.2451, -30.4003) (-8.1991, -30.4139) (-8.1683, -30.4225) (-8.1528, -30.4267) knots 0 0 0 0 0 0 0.0125 0.025 0.0375 0.05 0.0625 0.075 0.0875 0.1 0.1125 0.125 0.1375 0.15 0.1625 0.175 0.1875 0.2 0.2125 0.225 0.2375 0.25 0.2625 0.275 0.2875 0.3 0.3125 0.325 0.3375 0.35 0.3625 0.375 0.3875 0.4 0.4125 0.425 0.4375 0.45 0.4625 0.475 0.4875 0.5 0.5125 0.525 0.5375 0.55 0.5625 0.575 0.5875 0.6 0.6125 0.625 0.6375 0.65 0.6625 0.675 0.6875 0.7 0.7125 0.725 0.7375 0.75 0.7625 0.775 0.7875 0.8 0.8125 0.825 0.8375 0.85 0.8625 0.875 0.8875 0.9 0.9125 0.925 0.9375 0.95 0.9625 0.975 0.9875 1 1 1 1 1 1
  spline S34 degree 5 poles (-8.1528, -30.4267) (-8.1373, -30.4308) (-8.1063, -30.4388) (-8.0597, -30.45) (-7.9976, -30.4635) (-7.9199, -30.4778) (-7.8421, -30.4897) (-7.7642, -30.499) (-7.6864, -30.5058) (-7.6086, -30.5102) (-7.5311, -30.512) (-7.4539, -30.5114) (-7.3771, -30.5083) (-7.301, -30.5028) (-7.2258, -30.495) (-7.1515, -30.4848) (-7.0785, -30.4723) (-7.0067, -30.4578) (-6.9365, -30.4412) (-6.8679, -30.4226) (-6.8011, -30.4023) (-6.736, -30.3802) (-6.6729, -30.3565) (-6.6117, -30.3312) (-6.5525, -30.3044) (-6.4954, -30.2764) (-6.4405, -30.2472) (-6.388, -30.2173) (-6.3384, -30.1869) (-6.2917, -30.1565) (-6.2482, -30.1263) (-6.2078, -30.0967) (-6.1702, -30.0676) (-6.135, -30.0393) (-6.1019, -30.0117) (-6.0706, -29.9854) (-6.0416, -29.9613) (-6.0156, -29.9409) (-5.9939, -29.9256) (-5.9771, -29.9165) (-5.9651, -29.9129) (-5.9568, -29.9127) (-5.9502, -29.9139) (-5.9438, -29.9153) (-5.9361, -29.9186) (-5.9264, -29.9265) (-5.9144, -29.9415) (-5.9001, -29.9638) (-5.884, -29.9926) (-5.8664, -30.026) (-5.8476, -30.0623) (-5.8275, -30.1004) (-5.8059, -30.1401) (-5.7823, -30.1813) (-5.7563, -30.2242) (-5.7276, -30.2687) (-5.6961, -30.3147) (-5.6619, -30.3617) (-5.6249, -30.4094) (-5.5853, -30.4574) (-5.5433, -30.5052) (-5.4988, -30.5525) (-5.4519, -30.5993) (-5.4027, -30.6454) (-5.3511, -30.6907) (-5.2971, -30.7351) (-5.2408, -30.7785) (-5.1823, -30.8207) (-5.1216, -30.8616) (-5.0589, -30.9011) (-4.9942, -30.9389) (-4.9277, -30.975) (-4.8595, -31.0092) (-4.7897, -31.0414) (-4.7186, -31.0715) (-4.6463, -31.0994) (-4.5728, -31.1252) (-4.4983, -31.1486) (-4.4228, -31.1698) (-4.3463, -31.1886) (-4.269, -31.2051) (-4.2065, -31.2164) (-4.1592, -31.2239) (-4.1275, -31.2284) (-4.1116, -31.2305) knots 0 0 0 0 0 0 0.0125 0.025 0.0375 0.05 0.0625 0.075 0.0875 0.1 0.1125 0.125 0.1375 0.15 0.1625 0.175 0.1875 0.2 0.2125 0.225 0.2375 0.25 0.2625 0.275 0.2875 0.3 0.3125 0.325 0.3375 0.35 0.3625 0.375 0.3875 0.4 0.4125 0.425 0.4375 0.45 0.4625 0.475 0.4875 0.5 0.5125 0.525 0.5375 0.55 0.5625 0.575 0.5875 0.6 0.6125 0.625 0.6375 0.65 0.6625 0.675 0.6875 0.7 0.7125 0.725 0.7375 0.75 0.7625 0.775 0.7875 0.8 0.8125 0.825 0.8375 0.85 0.8625 0.875 0.8875 0.9 0.9125 0.925 0.9375 0.95 0.9625 0.975 0.9875 1 1 1 1 1 1
  spline S35 degree 5 poles (-4.1116, -31.2305) (-4.0957, -31.2326) (-4.0639, -31.2364) (-4.0163, -31.2415) (-3.9529, -31.2467) (-3.874, -31.2508) (-3.7953, -31.2524) (-3.7169, -31.2515) (-3.6388, -31.2481) (-3.5612, -31.2423) (-3.484, -31.234) (-3.4076, -31.2233) (-3.3319, -31.2102) (-3.2572, -31.1949) (-3.1836, -31.1772) (-3.1113, -31.1574) (-3.0405, -31.1356) (-2.9713, -31.1118) (-2.9038, -31.0861) (-2.8382, -31.0588) (-2.7746, -31.0299) (-2.713, -30.9995) (-2.6535, -30.9678) (-2.5961, -30.9347) (-2.5409, -30.9004) (-2.4879, -30.8651) (-2.4373, -30.8291) (-2.3893, -30.7926) (-2.344, -30.756) (-2.3017, -30.7197) (-2.2624, -30.6842) (-2.2262, -30.6495) (-2.1928, -30.6158) (-2.1616, -30.583) (-2.1324, -30.5514) (-2.1048, -30.5212) (-2.0792, -30.4935) (-2.0561, -30.4699) (-2.0365, -30.452) (-2.0211, -30.4407) (-2.0097, -30.4356) (-2.0014, -30.4343) (-1.9948, -30.4346) (-1.9882, -30.4352) (-1.9801, -30.4375) (-1.9695, -30.4441) (-1.9557, -30.4573) (-1.9386, -30.4776) (-1.9188, -30.504) (-1.897, -30.5348) (-1.8736, -30.5683) (-1.8487, -30.6036) (-1.8221, -30.6401) (-1.7934, -30.6779) (-1.762, -30.717) (-1.7278, -30.7574) (-1.6905, -30.7988) (-1.6504, -30.841) (-1.6075, -30.8835) (-1.5621, -30.9258) (-1.5141, -30.9677) (-1.4639, -31.0089) (-1.4113, -31.0492) (-1.3565, -31.0884) (-1.2994, -31.1266) (-1.2401, -31.1636) (-1.1786, -31.1992) (-1.1151, -31.2334) (-1.0496, -31.2661) (-0.9822, -31.297) (-0.9131, -31.3261) (-0.8424, -31.3532) (-0.7704, -31.3782) (-0.6971, -31.401) (-0.6226, -31.4216) (-0.5472, -31.4398) (-0.471, -31.4558) (-0.3941, -31.4693) (-0.3164, -31.4804) (-0.2382, -31.4891) (-0.1594, -31.4954) (-0.0959, -31.4984) (-0.0481, -31.4996) (-0.016, -31.5) (0, -31.5) knots 0 0 0 0 0 0 0.0125 0.025 0.0375 0.05 0.0625 0.075 0.0875 0.1 0.1125 0.125 0.1375 0.15 0.1625 0.175 0.1875 0.2 0.2125 0.225 0.2375 0.25 0.2625 0.275 0.2875 0.3 0.3125 0.325 0.3375 0.35 0.3625 0.375 0.3875 0.4 0.4125 0.425 0.4375 0.45 0.4625 0.475 0.4875 0.5 0.5125 0.525 0.5375 0.55 0.5625 0.575 0.5875 0.6 0.6125 0.625 0.6375 0.65 0.6625 0.675 0.6875 0.7 0.7125 0.725 0.7375 0.75 0.7625 0.775 0.7875 0.8 0.8125 0.825 0.8375 0.85 0.8625 0.875 0.8875 0.9 0.9125 0.925 0.9375 0.95 0.9625 0.975 0.9875 1 1 1 1 1 1
  spline S36 degree 5 poles (0, -31.5) (0.016, -31.5) (0.0481, -31.4996) (0.0959, -31.4984) (0.1594, -31.4954) (0.2382, -31.4891) (0.3164, -31.4804) (0.3941, -31.4693) (0.471, -31.4558) (0.5472, -31.4398) (0.6226, -31.4216) (0.697, -31.401) (0.7704, -31.3781) (0.8424, -31.3531) (0.9131, -31.326) (0.9822, -31.297) (1.0496, -31.266) (1.1151, -31.2334) (1.1786, -31.1992) (1.2401, -31.1636) (1.2994, -31.1266) (1.3565, -31.0884) (1.4113, -31.0492) (1.4639, -31.0089) (1.5141, -30.9677) (1.5621, -30.9258) (1.6075, -30.8835) (1.6504, -30.841) (1.6906, -30.7988) (1.7278, -30.7574) (1.762, -30.717) (1.7934, -30.6779) (1.8221, -30.6401) (1.8487, -30.6036) (1.8736, -30.5683) (1.897, -30.5348) (1.9188, -30.504) (1.9386, -30.4776) (1.9557, -30.4573) (1.9695, -30.4441) (1.9801, -30.4375) (1.9882, -30.4352) (1.9948, -30.4346) (2.0014, -30.4343) (2.0097, -30.4356) (2.0211, -30.4407) (2.0365, -30.452) (2.0561, -30.4699) (2.0792, -30.4935) (2.1048, -30.5212) (2.1324, -30.5514) (2.1616, -30.583) (2.1928, -30.6158) (2.2262, -30.6495) (2.2624, -30.6842) (2.3017, -30.7197) (2.344, -30.756) (2.3893, -30.7926) (2.4373, -30.8291) (2.4879, -30.8652) (2.5409, -30.9004) (2.5961, -30.9347) (2.6535, -30.9677) (2.713, -30.9995) (2.7746, -31.0299) (2.8382, -31.0588) (2.9038, -31.0862) (2.9713, -31.1118) (3.0405, -31.1356) (3.1113, -31.1575) (3.1836, -31.1773) (3.2572, -31.1949) (3.3319, -31.2103) (3.4076, -31.2233) (3.484, -31.234) (3.5612, -31.2423) (3.6388, -31.2481) (3.7169, -31.2515) (3.7953, -31.2524) (3.874, -31.2508) (3.9529, -31.2467) (4.0163, -31.2415) (4.0639, -31.2364) (4.0957, -31.2326) (4.1116, -31.2305) knots 0 0 0 0 0 0 0.0125 0.025 0.0375 0.05 0.0625 0.075 0.0875 0.1 0.1125 0.125 0.1375 0.15 0.1625 0.175 0.1875 0.2 0.2125 0.225 0.2375 0.25 0.2625 0.275 0.2875 0.3 0.3125 0.325 0.3375 0.35 0.3625 0.375 0.3875 0.4 0.4125 0.425 0.4375 0.45 0.4625 0.475 0.4875 0.5 0.5125 0.525 0.5375 0.55 0.5625 0.575 0.5875 0.6 0.6125 0.625 0.6375 0.65 0.6625 0.675 0.6875 0.7 0.7125 0.725 0.7375 0.75 0.7625 0.775 0.7875 0.8 0.8125 0.825 0.8375 0.85 0.8625 0.875 0.8875 0.9 0.9125 0.925 0.9375 0.95 0.9625 0.975 0.9875 1 1 1 1 1 1
  spline S37 degree 5 poles (4.1116, -31.2305) (4.1275, -31.2284) (4.1592, -31.2239) (4.2065, -31.2165) (4.269, -31.2051) (4.3463, -31.1886) (4.4228, -31.1698) (4.4983, -31.1486) (4.5728, -31.1252) (4.6463, -31.0994) (4.7186, -31.0715) (4.7897, -31.0413) (4.8595, -31.0091) (4.9276, -30.9749) (4.9942, -30.9389) (5.0589, -30.901) (5.1216, -30.8616) (5.1823, -30.8207) (5.2408, -30.7785) (5.2971, -30.7351) (5.3511, -30.6907) (5.4027, -30.6454) (5.452, -30.5993) (5.4988, -30.5525) (5.5433, -30.5052) (5.5853, -30.4574) (5.6249, -30.4094) (5.6619, -30.3617) (5.6961, -30.3147) (5.7276, -30.2687) (5.7563, -30.2242) (5.7823, -30.1813) (5.8059, -30.1401) (5.8275, -30.1004) (5.8476, -30.0623) (5.8664, -30.026) (5.884, -29.9926) (5.9001, -29.9638) (5.9144, -29.9415) (5.9264, -29.9265) (5.9361, -29.9186) (5.9438, -29.9153) (5.9502, -29.9139) (5.9568, -29.9127) (5.9651, -29.9129) (5.9771, -29.9165) (5.9939, -29.9257) (6.0156, -29.9409) (6.0416, -29.9613) (6.0706, -29.9854) (6.1019, -30.0117) (6.135, -30.0393) (6.1702, -30.0676) (6.2078, -30.0967) (6.2482, -30.1263) (6.2917, -30.1565) (6.3384, -30.1869) (6.3881, -30.2173) (6.4405, -30.2472) (6.4954, -30.2764) (6.5525, -30.3044) (6.6117, -30.3312) (6.6729, -30.3565) (6.736, -30.3802) (6.8011, -30.4023) (6.8679, -30.4226) (6.9365, -30.4412) (7.0067, -30.4578) (7.0785, -30.4724) (7.1515, -30.4848) (7.2258, -30.495) (7.3011, -30.5029) (7.3771, -30.5084) (7.4539, -30.5115) (7.5311, -30.5121) (7.6086, -30.5102) (7.6864, -30.5058) (7.7642, -30.499) (7.8421, -30.4896) (7.9199, -30.4778) (7.9976, -30.4634) (8.0597, -30.45) (8.1063, -30.4388) (8.1373, -30.4308) (8.1528, -30.4267) knots 0 0 0 0 0 0 0.0125 0.025 0.0375 0.05 0.0625 0.075 0.0875 0.1 0.1125 0.125 0.1375 0.15 0.1625 0.175 0.1875 0.2 0.2125 0.225 0.2375 0.25 0.2625 0.275 0.2875 0.3 0.3125 0.325 0.3375 0.35 0.3625 0.375 0.3875 0.4 0.4125 0.425 0.4375 0.45 0.4625 0.475 0.4875 0.5 0.5125 0.525 0.5375 0.55 0.5625 0.575 0.5875 0.6 0.6125 0.625 0.6375 0.65 0.6625 0.675 0.6875 0.7 0.7125 0.725 0.7375 0.75 0.7625 0.775 0.7875 0.8 0.8125 0.825 0.8375 0.85 0.8625 0.875 0.8875 0.9 0.9125 0.925 0.9375 0.95 0.9625 0.975 0.9875 1 1 1 1 1 1
  spline S38 degree 5 poles (8.1528, -30.4267) (8.1683, -30.4225) (8.1991, -30.4139) (8.2451, -30.4003) (8.3056, -30.3809) (8.3801, -30.3545) (8.4534, -30.3259) (8.5255, -30.295) (8.5963, -30.262) (8.6658, -30.2269) (8.7339, -30.1897) (8.8005, -30.1506) (8.8654, -30.1096) (8.9285, -30.0668) (8.9898, -30.0223) (9.049, -29.9763) (9.106, -29.929) (9.1609, -29.8806) (9.2134, -29.8311) (9.2635, -29.7807) (9.3113, -29.7297) (9.3565, -29.678) (9.3993, -29.6259) (9.4397, -29.5734) (9.4776, -29.5206) (9.513, -29.4678) (9.546, -29.4151) (9.5764, -29.363) (9.6043, -29.3118) (9.6295, -29.2621) (9.6521, -29.2143) (9.6723, -29.1684) (9.6903, -29.1244) (9.7065, -29.0823) (9.7214, -29.0418) (9.7354, -29.0034) (9.7485, -28.968) (9.7607, -28.9374) (9.772, -28.9133) (9.7819, -28.897) (9.7905, -28.8879) (9.7977, -28.8835) (9.8039, -28.8813) (9.8102, -28.8793) (9.8185, -28.8783) (9.8308, -28.8804) (9.8487, -28.8873) (9.8722, -28.8995) (9.9006, -28.9164) (9.9326, -28.9365) (9.967, -28.9585) (10.0035, -28.9815) (10.042, -29.005) (10.0831, -29.0289) (10.127, -29.0531) (10.1741, -29.0773) (10.2243, -29.1014) (10.2775, -29.125) (10.3334, -29.1478) (10.3917, -29.1695) (10.452, -29.1899) (10.5142, -29.2087) (10.5781, -29.2258) (10.6438, -29.2411) (10.7112, -29.2545) (10.7801, -29.2659) (10.8505, -29.2754) (10.9223, -29.2827) (10.9954, -29.2878) (11.0694, -29.2905) (11.1444, -29.291) (11.22, -29.289) (11.2962, -29.2845) (11.3727, -29.2775) (11.4493, -29.268) (11.5259, -29.256) (11.6024, -29.2416) (11.6787, -29.2246) (11.7547, -29.2052) (11.8303, -29.1833) (11.9055, -29.1589) (11.9653, -29.1375) (12.01, -29.1203) (12.0397, -29.1083) (12.0545, -29.1022) knots 0 0 0 0 0 0 0.0125 0.025 0.0375 0.05 0.0625 0.075 0.0875 0.1 0.1125 0.125 0.1375 0.15 0.1625 0.175 0.1875 0.2 0.2125 0.225 0.2375 0.25 0.2625 0.275 0.2875 0.3 0.3125 0.325 0.3375 0.35 0.3625 0.375 0.3875 0.4 0.4125 0.425 0.4375 0.45 0.4625 0.475 0.4875 0.5 0.5125 0.525 0.5375 0.55 0.5625 0.575 0.5875 0.6 0.6125 0.625 0.6375 0.65 0.6625 0.675 0.6875 0.7 0.7125 0.725 0.7375 0.75 0.7625 0.775 0.7875 0.8 0.8125 0.825 0.8375 0.85 0.8625 0.875 0.8875 0.9 0.9125 0.925 0.9375 0.95 0.9625 0.975 0.9875 1 1 1 1 1 1
  spline S39 degree 5 poles (12.0545, -29.1022) (12.0693, -29.096) (12.0988, -29.0835) (12.1426, -29.0641) (12.2001, -29.0369) (12.2705, -29.001) (12.3394, -28.963) (12.4068, -28.923) (12.4728, -28.8811) (12.5371, -28.8372) (12.5997, -28.7915) (12.6606, -28.744) (12.7196, -28.6948) (12.7766, -28.6441) (12.8315, -28.5921) (12.8842, -28.5388) (12.9347, -28.4844) (12.9827, -28.4292) (13.0283, -28.3733) (13.0714, -28.3168) (13.1121, -28.26) (13.1502, -28.2029) (13.1859, -28.1456) (13.219, -28.0883) (13.2497, -28.031) (13.278, -27.974) (13.3038, -27.9174) (13.3271, -27.8618) (13.3481, -27.8075) (13.3666, -27.7549) (13.3828, -27.7045) (13.3968, -27.6564) (13.4089, -27.6104) (13.4195, -27.5665) (13.429, -27.5245) (13.4378, -27.4846) (13.4462, -27.4477) (13.4543, -27.4158) (13.4623, -27.3905) (13.47, -27.373) (13.4773, -27.3628) (13.4839, -27.3576) (13.4898, -27.3545) (13.4958, -27.3517) (13.5039, -27.3497) (13.5164, -27.3501) (13.535, -27.3546) (13.5599, -27.3637) (13.5903, -27.3767) (13.6246, -27.3924) (13.6616, -27.4098) (13.7007, -27.4278) (13.742, -27.4462) (13.7858, -27.4645) (13.8325, -27.4827) (13.8824, -27.5005) (13.9354, -27.5178) (13.9912, -27.5343) (14.0496, -27.5496) (14.1101, -27.5636) (14.1726, -27.5759) (14.2367, -27.5864) (14.3024, -27.595) (14.3695, -27.6016) (14.438, -27.6061) (14.5079, -27.6085) (14.5789, -27.6086) (14.651, -27.6065) (14.7241, -27.602) (14.7979, -27.5951) (14.8723, -27.5857) (14.947, -27.5739) (15.0219, -27.5595) (15.0968, -27.5426) (15.1716, -27.5232) (15.246, -27.5013) (15.32, -27.477) (15.3934, -27.4502) (15.4662, -27.4211) (15.5382, -27.3895) (15.6096, -27.3555) (15.6661, -27.3264) (15.7082, -27.3035) (15.7361, -27.2878) (15.75, -27.2798) knots 0 0 0 0 0 0 0.0125 0.025 0.0375 0.05 0.0625 0.075 0.0875 0.1 0.1125 0.125 0.1375 0.15 0.1625 0.175 0.1875 0.2 0.2125 0.225 0.2375 0.25 0.2625 0.275 0.2875 0.3 0.3125 0.325 0.3375 0.35 0.3625 0.375 0.3875 0.4 0.4125 0.425 0.4375 0.45 0.4625 0.475 0.4875 0.5 0.5125 0.525 0.5375 0.55 0.5625 0.575 0.5875 0.6 0.6125 0.625 0.6375 0.65 0.6625 0.675 0.6875 0.7 0.7125 0.725 0.7375 0.75 0.7625 0.775 0.7875 0.8 0.8125 0.825 0.8375 0.85 0.8625 0.875 0.8875 0.9 0.9125 0.925 0.9375 0.95 0.9625 0.975 0.9875 1 1 1 1 1 1
  spline S40 degree 5 poles (15.75, -27.2798) (15.7639, -27.2717) (15.7915, -27.2555) (15.8323, -27.2305) (15.8858, -27.1961) (15.9509, -27.1513) (16.0143, -27.1046) (16.0759, -27.0562) (16.1358, -27.006) (16.1938, -26.9541) (16.25, -26.9006) (16.3041, -26.8455) (16.3562, -26.7891) (16.4061, -26.7314) (16.4538, -26.6726) (16.4991, -26.6129) (16.542, -26.5524) (16.5824, -26.4914) (16.6203, -26.43) (16.6557, -26.3684) (16.6886, -26.3067) (16.7189, -26.2451) (16.7468, -26.1837) (16.7722, -26.1226) (16.7951, -26.0618) (16.8157, -26.0015) (16.8339, -25.9421) (16.8498, -25.8839) (16.8635, -25.8273) (16.875, -25.7728) (16.8844, -25.7207) (16.892, -25.6711) (16.8981, -25.624) (16.9028, -25.5791) (16.9068, -25.5362) (16.9103, -25.4954) (16.9138, -25.4578) (16.9177, -25.4251) (16.9223, -25.399) (16.9277, -25.3806) (16.9336, -25.3696) (16.9394, -25.3635) (16.9448, -25.3597) (16.9504, -25.3562) (16.9582, -25.3531) (16.9707, -25.3519) (16.9897, -25.3539) (17.0156, -25.3597) (17.0474, -25.3686) (17.0834, -25.3797) (17.1224, -25.3921) (17.1636, -25.4049) (17.2069, -25.4177) (17.2527, -25.4301) (17.3014, -25.442) (17.3532, -25.4532) (17.4079, -25.4635) (17.4654, -25.4725) (17.5253, -25.4801) (17.5872, -25.486) (17.6507, -25.4901) (17.7157, -25.4921) (17.7819, -25.4921) (17.8493, -25.4899) (17.9178, -25.4854) (17.9874, -25.4786) (18.0578, -25.4695) (18.1291, -25.458) (18.2009, -25.444) (18.2732, -25.4275) (18.3457, -25.4085) (18.4182, -25.387) (18.4906, -25.363) (18.5627, -25.3364) (18.6343, -25.3074) (18.7052, -25.276) (18.7754, -25.2423) (18.8447, -25.2061) (18.913, -25.1677) (18.9804, -25.127) (19.0467, -25.084) (19.0989, -25.0478) (19.1376, -25.0196) (19.1632, -25.0004) (19.176, -24.9906) knots 0 0 0 0 0 0 0.0125 0.025 0.0375 0.05 0.0625 0.075 0.0875 0.1 0.1125 0.125 0.1375 0.15 0.1625 0.175 0.1875 0.2 0.2125 0.225 0.2375 0.25 0.2625 0.275 0.2875 0.3 0.3125 0.325 0.3375 0.35 0.3625 0.375 0.3875 0.4 0.4125 0.425 0.4375 0.45 0.4625 0.475 0.4875 0.5 0.5125 0.525 0.5375 0.55 0.5625 0.575 0.5875 0.6 0.6125 0.625 0.6375 0.65 0.6625 0.675 0.6875 0.7 0.7125 0.725 0.7375 0.75 0.7625 0.775 0.7875 0.8 0.8125 0.825 0.8375 0.85 0.8625 0.875 0.8875 0.9 0.9125 0.925 0.9375 0.95 0.9625 0.975 0.9875 1 1 1 1 1 1
  spline S41 degree 5 poles (19.176, -24.9906) (19.1887, -24.9808) (19.2139, -24.9611) (19.2512, -24.931) (19.2997, -24.8899) (19.3584, -24.837) (19.4151, -24.7825) (19.4699, -24.7264) (19.5227, -24.6688) (19.5735, -24.6098) (19.6222, -24.5494) (19.6687, -24.4877) (19.713, -24.425) (19.7549, -24.3613) (19.7945, -24.2968) (19.8316, -24.2316) (19.8662, -24.1661) (19.8983, -24.1003) (19.9279, -24.0345) (19.955, -23.9688) (19.9795, -23.9034) (20.0016, -23.8384) (20.0212, -23.7738) (20.0384, -23.7099) (20.0532, -23.6466) (20.0657, -23.5842) (20.076, -23.5229) (20.0842, -23.4631) (20.0903, -23.4052) (20.0946, -23.3497) (20.0972, -23.2968) (20.0983, -23.2466) (20.0981, -23.1992) (20.097, -23.154) (20.0953, -23.1109) (20.0934, -23.0701) (20.092, -23.0324) (20.0916, -22.9994) (20.0928, -22.9729) (20.0957, -22.9539) (20.1001, -22.9422) (20.1051, -22.9355) (20.11, -22.931) (20.1151, -22.9268) (20.1224, -22.9227) (20.1346, -22.9199) (20.1537, -22.9194) (20.1801, -22.9217) (20.2128, -22.9264) (20.25, -22.9328) (20.2902, -22.9399) (20.3327, -22.9472) (20.3774, -22.9542) (20.4244, -22.9606) (20.4742, -22.9661) (20.527, -22.9704) (20.5827, -22.9735) (20.6409, -22.9749) (20.7012, -22.9746) (20.7633, -22.9724) (20.8268, -22.9681) (20.8915, -22.9617) (20.9571, -22.953) (21.0237, -22.942) (21.091, -22.9286) (21.1591, -22.9128) (21.2278, -22.8946) (21.2969, -22.8739) (21.3663, -22.8506) (21.4358, -22.8248) (21.5052, -22.7966) (21.5743, -22.7657) (21.643, -22.7325) (21.711, -22.6968) (21.7782, -22.6587) (21.8444, -22.6183) (21.9095, -22.5756) (21.9735, -22.5308) (22.0362, -22.4838) (22.0977, -22.4346) (22.1579, -22.3833) (22.2049, -22.3406) (22.2396, -22.3076) (22.2625, -22.2852) (22.2739, -22.2739) knots 0 0 0 0 0 0 0.0125 0.025 0.0375 0.05 0.0625 0.075 0.0875 0.1 0.1125 0.125 0.1375 0.15 0.1625 0.175 0.1875 0.2 0.2125 0.225 0.2375 0.25 0.2625 0.275 0.2875 0.3 0.3125 0.325 0.3375 0.35 0.3625 0.375 0.3875 0.4 0.4125 0.425 0.4375 0.45 0.4625 0.475 0.4875 0.5 0.5125 0.525 0.5375 0.55 0.5625 0.575 0.5875 0.6 0.6125 0.625 0.6375 0.65 0.6625 0.675 0.6875 0.7 0.7125 0.725 0.7375 0.75 0.7625 0.775 0.7875 0.8 0.8125 0.825 0.8375 0.85 0.8625 0.875 0.8875 0.9 0.9125 0.925 0.9375 0.95 0.9625 0.975 0.9875 1 1 1 1 1 1
  spline S42 degree 5 poles (22.2739, -22.2739) (22.2852, -22.2625) (22.3076, -22.2396) (22.3406, -22.2049) (22.3833, -22.1579) (22.4346, -22.0977) (22.4838, -22.0363) (22.5308, -21.9735) (22.5756, -21.9095) (22.6183, -21.8444) (22.6587, -21.7781) (22.6967, -21.7109) (22.7324, -21.643) (22.7657, -21.5743) (22.7965, -21.5052) (22.8248, -21.4358) (22.8506, -21.3663) (22.8738, -21.2969) (22.8946, -21.2278) (22.9128, -21.1591) (22.9286, -21.091) (22.942, -21.0237) (22.953, -20.9571) (22.9617, -20.8915) (22.9681, -20.8268) (22.9724, -20.7633) (22.9746, -20.7012) (22.9749, -20.6409) (22.9735, -20.5827) (22.9704, -20.527) (22.9661, -20.4742) (22.9606, -20.4244) (22.9542, -20.3774) (22.9472, -20.3327) (22.9399, -20.2902) (22.9328, -20.25) (22.9264, -20.2128) (22.9217, -20.1801) (22.9194, -20.1537) (22.9199, -20.1345) (22.9227, -20.1224) (22.9268, -20.1151) (22.931, -20.11) (22.9355, -20.1051) (22.9422, -20.1001) (22.9539, -20.0957) (22.9729, -20.0928) (22.9994, -20.0916) (23.0324, -20.092) (23.0701, -20.0934) (23.1109, -20.0953) (23.154, -20.097) (23.1992, -20.0981) (23.2467, -20.0983) (23.2968, -20.0972) (23.3497, -20.0946) (23.4052, -20.0903) (23.4631, -20.0842) (23.5229, -20.076) (23.5842, -20.0657) (23.6466, -20.0532) (23.7099, -20.0384) (23.7738, -20.0212) (23.8384, -20.0016) (23.9034, -19.9795) (23.9688, -19.955) (24.0345, -19.9279) (24.1004, -19.8984) (24.1661, -19.8663) (24.2317, -19.8316) (24.2968, -19.7945) (24.3613, -19.755) (24.425, -19.713) (24.4878, -19.6687) (24.5494, -19.6222) (24.6098, -19.5735) (24.6688, -19.5227) (24.7264, -19.4699) (24.7824, -19.4151) (24.837, -19.3583) (24.8899, -19.2996) (24.931, -19.2511) (24.9611, -19.2139) (24.9808, -19.1887) (24.9906, -19.176) knots 0 0 0 0 0 0 0.0125 0.025 0.0375 0.05 0.0625 0.075 0.0875 0.1 0.1125 0.125 0.1375 0.15 0.1625 0.175 0.1875 0.2 0.2125 0.225 0.2375 0.25 0.2625 0.275 0.2875 0.3 0.3125 0.325 0.3375 0.35 0.3625 0.375 0.3875 0.4 0.4125 0.425 0.4375 0.45 0.4625 0.475 0.4875 0.5 0.5125 0.525 0.5375 0.55 0.5625 0.575 0.5875 0.6 0.6125 0.625 0.6375 0.65 0.6625 0.675 0.6875 0.7 0.7125 0.725 0.7375 0.75 0.7625 0.775 0.7875 0.8 0.8125 0.825 0.8375 0.85 0.8625 0.875 0.8875 0.9 0.9125 0.925 0.9375 0.95 0.9625 0.975 0.9875 1 1 1 1 1 1